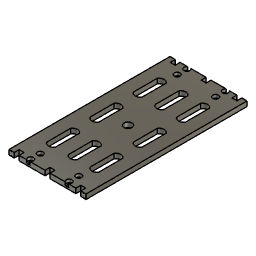
FS80+UL Pivot Base v12 (Autodesk Fusion 360 design; units mm, degrees)
Autodesk Fusion 360 part; units mm, degrees
sketch "Schizzo5" plane through (0, 0, 0) normal (0, 0, 1) x (1, 0, 0)
  line L0 (65.1728, 106.4816) -> (65.1728, -60.7184)
  circle A0 centre (85.1728, -58.2184) radius 1.5
  circle A1 centre (125.1728, 103.9816) radius 3
  line L1 (65.1728, 22.8816) -> (145.1728, 22.8816) construction
  circle A2 centre (85.1728, 103.9816) radius 3
  circle A3 centre (85.1728, 103.9816) radius 1.5
  line L2 (145.1728, 106.4816) -> (65.1728, 106.4816)
  circle A4 centre (125.1728, 103.9816) radius 1.5
  line L3 (105.1728, 25.3816) -> (105.1728, 1.3102) construction
  circle A5 centre (105.1728, 22.8816) radius 4.1
  line L4 (145.1728, -60.7184) -> (145.1728, 106.4816)
  line L5 (85.1728, 106.4816) -> (85.1728, -60.7184) construction
  circle A6 centre (85.1728, -58.2184) radius 3
  circle A7 centre (125.1728, -58.2184) radius 1.5
  line L6 (65.1728, -60.7184) -> (145.1728, -60.7184)
  circle A8 centre (125.1728, -58.2184) radius 3
  line L7 (65.1728, -58.2184) -> (145.1728, -58.2184) construction
  line L8 (105.1728, 106.4816) -> (105.1728, -60.7184) construction
  line L9 (105.1728, 25.3816) -> (105.1728, 56.9762) construction
  line L10 (105.1728, 25.3816) -> (105.1728, 56.9762) construction
  line L11 (105.1728, 25.3816) -> (105.1728, 1.3102) construction
  line L12 (65.1728, -48.2184) -> (145.1728, -48.2184) construction
  circle A9 centre (85.1728, -48.2184) radius 1.5
  circle A10 centre (85.1728, -48.2184) radius 3
  circle A11 centre (125.1728, -48.2184) radius 3
  circle A12 centre (125.1728, -48.2184) radius 1.5
  circle A13 centre (85.1728, 93.9816) radius 3
  circle A14 centre (85.1728, 93.9816) radius 1.5
  circle A15 centre (125.1728, 93.9816) radius 3
  circle A16 centre (125.1728, 93.9816) radius 1.5
  line L13 (107.7228, -60.7184) -> (102.6228, -60.7184)
  line L14 (102.6228, -60.7184) -> (102.6228, -55.6184)
  line L15 (102.6228, -55.6184) -> (107.7228, -55.6184)
  line L16 (107.7228, -55.6184) -> (107.7228, -60.7184)
  line L17 (107.7228, -60.7184) -> (102.6228, -55.6184) construction
  line L18 (102.6228, -60.7184) -> (107.7228, -55.6184) construction
  line L19 (102.6228, 101.3816) -> (107.7228, 101.3816)
  line L20 (102.6228, 106.4816) -> (102.6228, 101.3816)
  line L21 (107.7228, 101.3816) -> (107.7228, 106.4816)
  line L22 (70.6228, -55.6184) -> (75.7228, -55.6184)
  line L23 (75.7228, -55.6184) -> (75.7228, -60.7184)
  line L24 (75.7228, -60.7184) -> (70.6228, -60.7184)
  line L25 (70.6228, -60.7184) -> (70.6228, -55.6184)
  line L26 (134.6228, -55.6184) -> (134.6228, -60.7184)
  line L27 (139.7228, -55.6184) -> (134.6228, -55.6184)
  line L28 (139.7228, -60.7184) -> (139.7228, -55.6184)
  line L29 (134.6228, -60.7184) -> (139.7228, -60.7184)
  line L30 (70.6228, -60.7184) -> (75.7228, -55.6184) construction
  line L31 (70.6228, -55.6184) -> (75.7228, -60.7184) construction
  line L32 (70.6228, 101.3816) -> (75.7228, 101.3816)
  line L33 (75.7228, 101.3816) -> (75.7228, 106.4816)
  line L34 (70.6228, 106.4816) -> (70.6228, 101.3816)
  line L35 (75.7228, 106.4816) -> (70.6228, 106.4816)
  line L36 (139.7228, 101.3816) -> (134.6228, 101.3816)
  line L37 (134.6228, 101.3816) -> (134.6228, 106.4816)
  line L38 (139.7228, 106.4816) -> (139.7228, 101.3816)
  line L39 (134.6228, 106.4816) -> (139.7228, 106.4816)
  line L40 (78.1728, 35.3816) -> (87.1728, 35.3816)
  line L41 (87.1728, 35.3816) -> (87.1728, 10.3816)
  line L42 (87.1728, 10.3816) -> (78.1728, 10.3816)
  line L43 (78.1728, 10.3816) -> (78.1728, 35.3816)
  arc A17 (78.1728, 10.3816) -> (87.1728, 10.3816) centre (82.6728, 13.1816) ccw
  line L44 (78.1728, 22.8816) -> (87.1728, 22.8816) construction
  arc A18 (87.1728, 35.3816) -> (78.1728, 35.3816) centre (82.6728, 32.5816) ccw
  arc A19 (132.1728, 35.3816) -> (123.1728, 35.3816) centre (127.6728, 32.5816) ccw
  line L45 (132.1728, 35.3816) -> (123.1728, 35.3816)
  line L46 (123.1728, 35.3816) -> (123.1728, 10.3816)
  line L47 (132.1728, 10.3816) -> (132.1728, 35.3816)
  line L48 (123.1728, 10.3816) -> (132.1728, 10.3816)
  arc A20 (123.1728, 10.3816) -> (132.1728, 10.3816) centre (127.6728, 13.1816) ccw
  line L49 (82.6728, 35.3816) -> (82.6728, 10.3816) construction
  line L50 (127.6728, 35.3816) -> (127.6728, 10.3816) construction
  line L51 (132.1728, 22.8816) -> (123.1728, 22.8816) construction
  line L52 (109.6728, -34.6184) -> (100.6728, -34.6184)
  line L53 (100.6728, -34.6184) -> (100.6728, -9.6184)
  line L54 (100.6728, -9.6184) -> (109.6728, -9.6184)
  line L55 (109.6728, -9.6184) -> (109.6728, -34.6184)
  line L56 (109.6728, -34.6184) -> (100.6728, -9.6184) construction
  line L57 (100.6728, -34.6184) -> (109.6728, -9.6184) construction
  arc A21 (109.6728, -9.6184) -> (100.6728, -9.6184) centre (105.1728, -12.4184) ccw
  line L58 (100.6728, -22.1184) -> (109.6728, -22.1184) construction
  arc A22 (100.6728, -34.6184) -> (109.6728, -34.6184) centre (105.1728, -31.8184) ccw
  line L59 (82.6728, 37.8816) -> (82.6728, 35.3816) construction
  arc A23 (100.6728, 55.3816) -> (109.6728, 55.3816) centre (105.1728, 58.1816) ccw
  line L60 (109.6728, 55.3816) -> (109.6728, 80.3816)
  line L61 (100.6728, 80.3816) -> (100.6728, 55.3816)
  arc A24 (109.6728, 80.3816) -> (100.6728, 80.3816) centre (105.1728, 77.5816) ccw
  line L62 (100.6728, 80.3816) -> (109.6728, 55.3816) construction
  line L63 (109.6728, 80.3816) -> (100.6728, 55.3816) construction
  line L64 (78.1728, -9.6184) -> (87.1728, -9.6184)
  line L65 (87.1728, -9.6184) -> (87.1728, -34.6184)
  line L66 (87.1728, -34.6184) -> (78.1728, -34.6184)
  line L67 (78.1728, -34.6184) -> (78.1728, -9.6184)
  line L68 (82.6728, -9.6184) -> (82.6728, -34.6184) construction
  line L69 (78.1728, -22.1184) -> (87.1728, -22.1184) construction
  line L70 (82.6728, -9.6184) -> (82.6728, -7.1184) construction
  arc A25 (87.1728, -9.6184) -> (78.1728, -9.6184) centre (82.6728, -12.4184) ccw
  arc A26 (78.1728, -34.6184) -> (87.1728, -34.6184) centre (82.6728, -31.8184) ccw
  arc A27 (132.1728, -9.6184) -> (123.1728, -9.6184) centre (127.6728, -12.4184) ccw
  line L71 (132.1728, -34.6184) -> (132.1728, -9.6184)
  line L72 (123.1728, -9.6184) -> (123.1728, -34.6184)
  arc A28 (123.1728, -34.6184) -> (132.1728, -34.6184) centre (127.6728, -31.8184) ccw
  line L73 (82.6728, 13.1816) -> (82.6728, -60.7184) construction
  arc A29 (78.1728, 55.3816) -> (87.1728, 55.3816) centre (82.6728, 58.1816) ccw
  line L74 (78.1728, 80.3816) -> (78.1728, 55.3816)
  line L75 (87.1728, 55.3816) -> (87.1728, 80.3816)
  arc A30 (87.1728, 80.3816) -> (78.1728, 80.3816) centre (82.6728, 77.5816) ccw
  arc A31 (132.1728, 80.3816) -> (123.1728, 80.3816) centre (127.6728, 77.5816) ccw
  line L76 (132.1728, 80.3816) -> (132.1728, 55.3816)
  line L77 (123.1728, 55.3816) -> (123.1728, 80.3816)
  arc A32 (123.1728, 55.3816) -> (132.1728, 55.3816) centre (127.6728, 58.1816) ccw
  point P0 (105.1728, -58.1684)
  point P1 (105.1728, 25.3816)
  point P2 (73.1728, -58.1684)
  point P3 (82.6728, 22.8816)
  point P4 (127.6728, 22.8816)
  point P5 (105.1728, -22.1184)
  point P6 (105.1728, -7.1184)
  point P7 (105.1728, 67.8816)
  dimension "d221" = 80
  dimension "d222" = 167.2
  dimension "d223" = 2.5
  dimension "d224" = 20
  dimension "d225" = 3
  dimension "d226" = 6
  dimension "d229" = 8.2
  dimension "d350" = 3
  dimension "d351" = 6
  dimension "d354" = 10
  dimension "d355" = 5.1
  dimension "d356" = 5.1
  dimension "d368" = 5.1
  dimension "d369" = 5.1
  dimension "d370" = 32
  dimension "d371" = 9
  dimension "d372" = 25
  dimension "d373" = 45
  dimension "d380" = 9
  dimension "d381" = 25
  dimension "d382" = 2.5
  dimension "d383" = 2.5
  dimension "d384" = 90
  dimension "d385" = 9
  dimension "d386" = 25
  dimension "d387" = 2.5
  constraint horizontal L6
  constraint vertical L4
  constraint horizontal L2
  constraint vertical L0
  constraint midpoint L8.start L2
  constraint midpoint L8.end L6
  constraint coincident L7.end L4
  constraint perpendicular L4 L7
  constraint midpoint L1.start L0
  constraint midpoint L1.end L4
  constraint coincident L5.start L2
  constraint coincident L5.end L6
  constraint perpendicular L5 L6
  constraint coincident A0.centre L7
  constraint coincident A0.centre L5
  constraint concentric A0 A6
  constraint symmetric A0 A7 L8
  constraint symmetric A6 A8 L8
  constraint symmetric A0 L1 A3
  constraint symmetric L1 A2 A6
  constraint symmetric L1 A4 A7
  constraint symmetric A1 L1 A8
  constraint midpoint A5.centre L1
  constraint coincident L3.end L8
  constraint coincident P1 L3.start
  constraint coincident L9.end L8
  constraint coincident L7.start L0
  constraint coincident L0 L12.start
  constraint coincident L4 L12.end
  constraint perpendicular L4 L12
  constraint coincident L12 A9.centre
  constraint coincident L5 A9.centre
  constraint concentric A9 A10
  constraint symmetric L8 A9 A12
  constraint symmetric L8 A10 A11
  constraint symmetric L1 A9 A14
  constraint symmetric L1 A10 A13
  constraint symmetric L1 A11 A15
  constraint symmetric L1 A12 A16
  constraint horizontal L13
  constraint perpendicular L13 L14
  constraint parallel L13 L15
  constraint parallel L14 L16
  constraint coincident L17 P0
  constraint coincident L18 P0
  constraint coincident L8 P0
  constraint collinear L6 L13
  constraint symmetric L1 L13.start L21.end
  constraint symmetric L1 L13.end L20.start
  constraint symmetric L1 L14.end L19.start
  constraint symmetric L1 L15.end L19.end
  constraint horizontal L22
  constraint vertical L23
  constraint horizontal L24
  constraint vertical L25
  constraint symmetric L8 L22.start L27.start
  constraint symmetric L8 L22.end L26.start
  constraint symmetric L8 L23.end L26.end
  constraint symmetric L8 L24.end L28.start
  constraint collinear L6 L24
  constraint midpoint L30 P2
  constraint symmetric L1 L22.start L32.start
  constraint symmetric L1 L22.end L32.end
  constraint symmetric L1 L23.end L33.end
  constraint symmetric L1 L24.end L34.start
  constraint symmetric L1 L26.start L36.end
  constraint symmetric L1 L26.end L37.end
  constraint symmetric L1 L27.start L36.start
  constraint symmetric L1 L28.start L38.start
  constraint horizontal L40
  constraint vertical L41
  constraint horizontal L42
  constraint vertical L43
  constraint midpoint L43 L44.start
  constraint midpoint L41 L44.end
  constraint symmetric L41.end L44 L40.end
  constraint symmetric L42.end L44 L40.start
  constraint symmetric A17 L44 A18
  constraint symmetric L8 L40.start A19.start
  constraint symmetric L8 L40.end A19.end
  constraint symmetric L8 L41.end L46.end
  constraint symmetric L8 L42.end L47.start
  constraint symmetric L8 A17 A20
  constraint symmetric L8 A18 A19
  constraint midpoint L40 L49.start
  constraint midpoint L42 L49.end
  constraint midpoint L44 P3
  constraint symmetric L8 L44.start L51.start
  constraint symmetric L8 L44.end L51.end
  constraint symmetric L8 L49.start L50.start
  constraint symmetric L8 L49.end L50.end
  constraint symmetric L8 P3 P4
  constraint collinear L1 L44
  constraint horizontal L52
  constraint perpendicular L52 L53
  constraint parallel L52 L54
  constraint parallel L53 L55
  constraint coincident L56 P5
  constraint coincident L57 P5
  constraint coincident L8 P5
  constraint midpoint L53 L58.start
  constraint midpoint L55 L58.end
  constraint symmetric L53.end L58 L52.end
  constraint symmetric L54.end L58 L52.start
  constraint symmetric A21 L58 A22
  constraint midpoint A21 P6
  constraint midpoint A18 L59.start
  constraint symmetric L1 L52.start L60.end
  constraint symmetric L1 L52.end L61.start
  constraint symmetric L1 L53.end A23.start
  constraint symmetric L1 L54.end A23.end
  constraint symmetric L1 A21 A23
  constraint symmetric L1 A22 A24
  constraint symmetric L1 P5 P7
  constraint horizontal L64
  constraint vertical L65
  constraint horizontal L66
  constraint vertical L67
  constraint midpoint L64 L68.start
  constraint midpoint L66 L68.end
  constraint midpoint L67 L69.start
  constraint midpoint L65 L69.end
  constraint perpendicular L64 L70
  constraint coincident L70.end A25
  constraint symmetric L64.start L69 L66.end
  constraint symmetric L64.end L69 L65.end
  constraint symmetric L69 A25 A26
  constraint symmetric L8 L64.start A27.start
  constraint symmetric L8 L64.end A27.end
  constraint symmetric L8 L65.end L72.end
  constraint symmetric L8 L66.end L71.start
  constraint symmetric L8 A25 A27
  constraint symmetric L8 A26 A28
  constraint coincident A17.centre L73.start
  constraint coincident L6 L73.end
  constraint perpendicular L6 L73
  constraint collinear L68 L73
  constraint collinear L58 L69
  constraint symmetric L1 L64.start A29.start
  constraint symmetric L1 L64.end A29.end
  constraint symmetric L1 L65.end L75.end
  constraint symmetric L1 L66.end L74.start
  constraint symmetric L1 A25 A29
  constraint symmetric L1 A26 A30
  constraint symmetric L1 A27.end L77.start
  constraint symmetric L1 A27.start L76.end
  constraint symmetric L1 A27 A32
  constraint symmetric L1 L71.start A31.start
  constraint symmetric L1 L72.end A31.end
  constraint symmetric L1 A28 A31
  measures "d221" distance of L0.end L4.start
  measures "d222" distance of L0.end L0.start
  measures "d223" distance of L6 L7
  measures "d224" distance of L5 L8
  measures "d225" diameter of A0
  measures "d226" diameter of A6
  measures "d229" diameter of A5
  measures "d350" diameter of A9
  measures "d351" diameter of A10
  measures "d354" distance of L7 L12
  measures "d355" distance of L14.end L15.end
  measures "d356" distance of L13.end L14.end
  measures "d368" distance of L22.start L22.end
  measures "d369" distance of L22.start L24.end
  measures "d370" distance of L8 P2
  measures "d371" distance of L40.start L40.end
  measures "d372" distance of L40.start L42.end
  measures "d373" distance of L49 L50
  measures "d380" distance of L53.end L54.end
  measures "d381" distance of L52.end L53.end
  measures "d382" distance of L54 P6
  measures "d383" distance of L40 L59.start
  measures "d384" distance of P5 P7
  measures "d385" distance of L64.start L64.end
  measures "d386" distance of L64.start L66.end
  measures "d387" distance of L64 L70.end
extrude "Estrusione24" add sketch "Schizzo5" along normal blind 5 contours L0 A1 A2 L2 L4 A6 L6 A8 L14 L15 L16 L19 L20 L21 L22 L23 L25 L26 L27 L28 L32 L33 L34 L36 L37 L38
extrude "Estrusione25" add sketch "Schizzo5" along normal blind 1.8 contours A2 L2 | A6 L6 | A1 L2 | L6 A8 | A10 | A11 | A13 | A15 picked at (85.2101, 106.1469) picked at (85.2101, -60.3837) picked at (125.2101, 106.1469) picked at (125.2101, -60.3837)
sketch "Schizzo17" plane through (0, -60.7184, 0) normal (0, -1, 0) x (1, 0, 0)
  line L0 (75.7228, 0) -> (102.6228, 0)
  line L1 (102.6228, 0) -> (102.6228, 5)
  line L2 (102.6228, 5) -> (86.8311, 5)
  line L3 (86.8311, 5) -> (86.8311, 1.8)
  line L4 (86.8311, 1.8) -> (83.5144, 1.8)
  line L5 (83.5144, 1.8) -> (83.5144, 5)
  line L6 (65.1728, 5) -> (145.1728, 5) construction
  line L7 (145.1728, 5) -> (145.1728, 0) construction
  line L8 (145.1728, 0) -> (65.1728, 0) construction
  line L9 (65.1728, 0) -> (65.1728, 5) construction
  line L10 (107.7228, 0) -> (134.6228, 0) construction
  line L11 (107.7228, 5) -> (123.5144, 5) construction
  line L12 (145.1728, 0) -> (145.1728, 5) construction
  line L13 (65.1728, 2.5) -> (145.1728, 2.5) construction
  line L14 (77.9024, 5) -> (-23.8923, 0) construction
  circle A0 centre (67.723, 4.5) radius 0.4
  circle A1 centre (67.723, 0.5) radius 0.4
  line L15 (105.1728, 5) -> (105.1728, 0) construction
  line L16 (132.4431, 5) -> (234.2378, 0) construction
  circle A2 centre (142.6225, 0.5) radius 0.4
  circle A3 centre (142.6225, 4.5) radius 0.4
  line L17 (83.5144, 5) -> (75.7228, 5)
  line L18 (75.7228, 5) -> (75.7228, 0)
  line L19 (139.7228, 0) -> (145.1728, 0)
  point P0 (142.6225, 4.5)
  point P1 (142.6225, 0.5)
  point P2 (142.6225, 4.5)
  dimension "d357" = 0.8
  dimension "d358" = 4
  constraint horizontal L6
  constraint vertical L7
  constraint horizontal L8
  constraint vertical L9
  constraint collinear L8 L10
  constraint collinear L6 L11
  constraint collinear L7 L12
  constraint midpoint L7 L13.end
  constraint coincident L6 L14.start
  constraint coincident L8 L14.end
  constraint coincident L14 A0.centre
  constraint symmetric L13 A0 A1
  constraint midpoint L6 L15.start
  constraint midpoint L8 L15.end
  constraint symmetric L14.start L15 L16.start
  constraint symmetric L14.end L15 L16.end
  constraint symmetric A0.centre L15 P2
  constraint symmetric A1.centre L15 P1
  constraint symmetric A1 L15 A2
  constraint symmetric A0 L15 A3
  measures "d357" diameter of A0
  measures "d358" distance of A0.centre A1.centre
extrude "Estrusione29" cut sketch "Schizzo17" against normal blind 180 contours A0 | A1 | A2 | A3
equation "d225 = d227"
equation "d226 = d228"
equation "d227 = 3.00 mm"
equation "d228 = 6.00 mm"
equation "d350 = d227"
equation "d351 = d228"
equation "d355 = d356"
equation "d368 = d356"
equation "d369 = d356"
named bodies: "Base"
